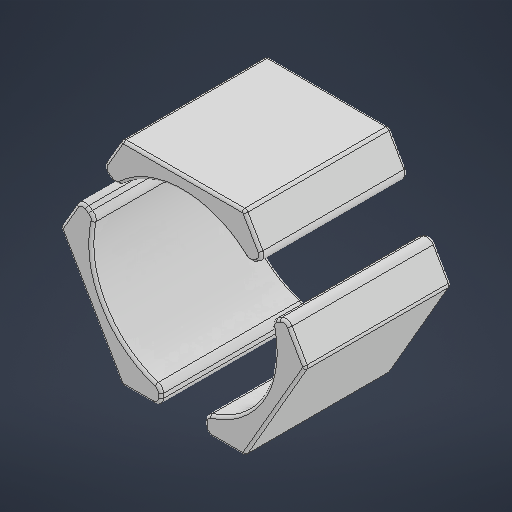
# Autodesk Inventor part: wheel holding tools
Saved by Autodesk Inventor 2027 (Build 310192000, 192)
## iProperties
Created: 2026-04-14
Part Number: wheel holding tools
Material: Všeobecné
Document SubType Name: Modeling
Designer: Vadim
Density: 1 g/cm^3
Appearance: Výchozí
Author: Vadim
Autodesk Inventor part; units mm, degrees
ref_plane "YZ Plane" through (0, 0, 0) normal (1, 0, 0) x (0, 1, 0)
ref_plane "XZ Plane" through (0, 0, 0) normal (0, 1, 0) x (-1, 0, 0)
ref_plane "XY Plane" through (0, 0, 0) normal (0, 0, 1) x (1, 0, 0)
sketch "Náčrt1" plane through (0, 0, 0) normal (0, 0, 1) x (1, 0, 0)
  circle A0 centre (0, 0) radius 12.55
  line L0 (8.4004, 14.55) -> (16.8009, 0)
  line L1 (16.8009, 0) -> (8.4004, -14.55)
  line L2 (8.4004, -14.55) -> (-8.4004, -14.55)
  line L3 (-8.4004, -14.55) -> (-16.8009, 0)
  line L4 (-16.8009, 0) -> (-8.4004, 14.55)
  line L5 (-8.4004, 14.55) -> (8.4004, 14.55)
  circle A1 centre (0, 0) radius 14 construction
  line L6 (-12.6007, 7.275) -> (0, 0)
  line L7 (0, 0) -> (0, -14.55)
  line L8 (-11.2676, 9.9695) -> (1.4776, 2.611)
  line L9 (-14.5304, 4.925) -> (-1.5224, -2.5851)
  line L10 (-3, -0.05) -> (-3, -14.55)
  line L11 (3, -0.05) -> (3, -14.55)
  line L12 (0, 14.55) -> (0, 0) construction
  line L13 (11.2676, 9.9695) -> (-1.4776, 2.611)
  line L14 (14.5304, 4.925) -> (1.5224, -2.5851)
  point P0 (14.1007, 4.6769)
  point P1 (12.0535, 3.495)
  point P2 (3, -12.1862)
  point P3 (3, -14.55)
  point P4 (-3, -14.55)
  point P5 (-3, -12.1862)
  point P6 (-12.0535, 3.495)
  point P7 (-14.1007, 4.6769)
  point P8 (-11.1007, 9.8731)
  point P9 (-9.0535, 8.6912)
  point P10 (9.0535, 8.6912)
  point P11 (11.1007, 9.8731)
  dimension "d0" = 25.1
  dimension "d1" = 14.55
  dimension "d2" = 28
  dimension "d4" = 3
  dimension "d5" = 3
  dimension "d6" = 3
  dimension "d7" = 3
  constraints: 30 end point, 5 symmetric about line, 4 parallel, 3 coincident, 3 midpoint, 2 centre point, 1 vertical, 13 other
  measures "d0" diameter of A0
  measures "d1" distance from line of A0.centre L5
  measures "d2" diameter of A1
  measures "d4" distance between parallel lines of L6 L8
  measures "d5" distance between parallel lines of L6 L9
  measures "d6" distance between parallel lines of L7 L10
  measures "d7" distance between parallel lines of L7 L11
extrude "Vysunutí1" add sketch "Náčrt1" along normal blind 20 contours A0 L14 L0 L1 L2 L11 | A0 L8 L4 L5 L0 L13 | L10 L2 L3 L4 L9 A0
fillet "Zaoblení1" radius 1 12 edges at (-12.0535, 3.495, 10) (-9.0535, 8.6912, 10) (-11.1007, 9.8731, 10) (-14.1007, 4.6769, 10) (11.1007, 9.8731, 10) (9.0535, 8.6912, 10) (14.1007, 4.6769, 10) (12.0535, 3.495, 10) (3, -12.1862, 10) (3, -14.55, 10) (-3, -12.1862, 10) (-3, -14.55, 10)
fillet "Zaoblení1" radius 0.5 6 edges at (-16.8009, 0, 10) (-8.4004, -14.55, 10) (-8.4004, 14.55, 10) (8.4004, 14.55, 10) (16.8009, 0, 10) (8.4004, -14.55, 10)
fillet "Zaoblení1" radius 0.35 36 edges at (-15.4508, 2.3385, 20) (-13.0771, 4.086, 20) (-10.8686, -6.275, 20) (-12.6007, -7.275, 20) (-3, -13.3681, 20) (-5.7002, -14.55, 20) (10.8686, -6.275, 20) (3, -13.3681, 20) (5.7002, -14.55, 20) (12.6007, -7.275, 20) (15.4508, 2.3385, 20) (13.0771, 4.086, 20) (0, 12.55, 20) (10.0771, 9.2821, 20) (9.7506, 12.2115, 20) (0, 14.55, 20) (-9.7506, 12.2115, 20) (-10.0771, 9.2821, 20) (0, 12.55, 0) (0, 14.55, 0) (-9.7506, 12.2115, 0) (-10.0771, 9.2821, 0) (9.7506, 12.2115, 0) (10.0771, 9.2821, 0) (13.0771, 4.086, 0) (15.4508, 2.3385, 0) (10.8686, -6.275, 0) (12.6007, -7.275, 0) (5.7002, -14.55, 0) (3, -13.3681, 0) (-3, -13.3681, 0) (-5.7002, -14.55, 0) (-10.8686, -6.275, 0) (-12.6007, -7.275, 0) (-13.0771, 4.086, 0) (-15.4508, 2.3385, 0)
equation "\"d5\" = d4"
equation "\"d6\" = d4"
equation "\"d7\" = d4"
